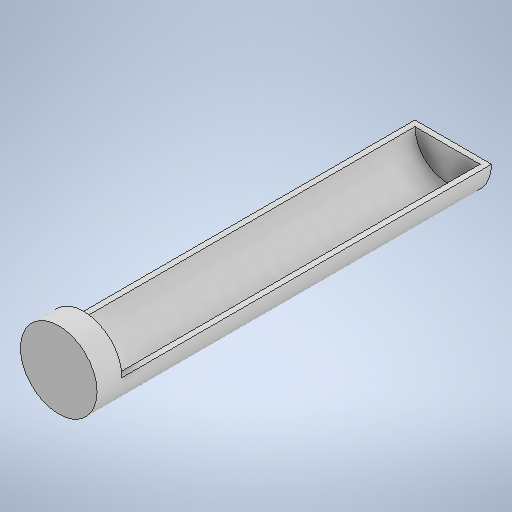
# Autodesk Inventor part: prototype3
Saved by Autodesk Inventor 2025.1 (Build 291241020, 241B)
## iProperties
Created: 2024-11-22
Part Number: prototype3
Material: Generic
Document SubType Name: Modeling
Designer: leon-
Density: 1 g/cm^3
Appearance: Default
Author: leon-
Autodesk Inventor part; units mm, degrees
ref_plane "YZ Plane" through (0, 0, 0) normal (1, 0, 0) x (0, 1, 0)
ref_plane "XZ Plane" through (0, 0, 0) normal (0, 1, 0) x (-1, 0, 0)
ref_plane "XY Plane" through (0, 0, 0) normal (0, 0, 1) x (1, 0, 0)
sketch "Sketch1" plane through (0, 0, 0) normal (0, 0, 1) x (1, 0, 0)
  arc A0 (-17, 0) -> (17, 0) centre (0, 0) ccw
  line L0 (-23.8, 0) -> (23.8, 0) projected
  line L1 (-17, 0) -> (17, 0)
  dimension "d1" = 17
  constraints: 2 end point, 2 point on circle, 2 point on line, 1 centre point, 1 coincident, 1 collinear
  measures "d1" radius of A0
extrude "Extrusion1" add sketch "Sketch1" along normal blind 200
shell "Shell1" thickness 3 outward yes removed faces 1 at (5.6667, 0, 66.6667)
sketch "Sketch2" plane through (0, 0, 200) normal (0, 0, -1) x (-1, 0, 0)
  circle A0 centre (0, 0) radius 20
  arc A1 (-20, 0) -> (20, 0) centre (0, 0) ccw projected
  constraints: 2 concentric, 1 centre point, 1 coincident
extrude "Extrusion2" add sketch "Sketch2" against normal up to surface (3 mm away)
sketch "Sketch3" plane through (0, 0, 200) normal (0, 0, -1) x (-1, 0, 0)
  circle A0 centre (0, 0) radius 11
  circle A1 centre (0, 0) radius 20
  circle A2 centre (0, 0) radius 20 projected
  dimension "d7" = 22
  constraints: 2 centre point, 2 coincident, 1 concentric
  measures "d7" diameter of A0
extrude "Extrusion3" add sketch "Sketch3" along normal blind 10
body "Solid1"
